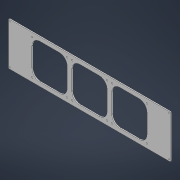
# Autodesk Inventor part: radiator_adapter_03
Saved by Autodesk Inventor 2022 (Build 260153000, 153)
## iProperties
Created: 2025-02-08
Part Number: radiator_adapter_03
Material: 一般
Document SubType Name: Modeling
Designer: gisen
Density: 1 g/cm^3
Appearance: 既定
Author: gisen
Autodesk Inventor part; units mm, degrees
ref_plane "YZ Plane" through (0, 0, 0) normal (1, 0, 0) x (0, 1, 0)
ref_plane "XZ Plane" through (0, 0, 0) normal (0, 1, 0) x (-1, 0, 0)
ref_plane "XY Plane" through (0, 0, 0) normal (0, 0, 1) x (1, 0, 0)
sketch "スケッチ1" plane through (0, 0, 0) normal (0, 0, 1) x (1, 0, 0)
  circle A0 centre (5, 125) radius 2.25 construction
  circle A1 centre (5, 5) radius 2.25 construction
  circle A2 centre (-473, 125) radius 2.25 construction
  circle A3 centre (-473, 5) radius 2.25 construction
  line L0 (-478, 130) -> (-478, 0) construction
  line L1 (10, 0) -> (10, 130) construction
  line L2 (10, 130) -> (-478, 130)
  line L3 (-478, 130) -> (-478, 0)
  line L4 (-478, 0) -> (10, 0)
  line L5 (10, 0) -> (10, 130)
  circle A4 centre (5, 125) radius 1.6
  circle A5 centre (5, 5) radius 1.6
  circle A6 centre (-473, 5) radius 1.6
  circle A7 centre (-473, 125) radius 1.6
  line L6 (10, 65) -> (-478, 65) construction
  line L7 (-205, 118) -> (-263, 118)
  line L8 (-287, 94) -> (-287, 36)
  line L9 (-263, 12) -> (-205, 12)
  line L10 (-181, 36) -> (-181, 94)
  arc A8 (-181, 94) -> (-205, 118) centre (-205, 94) ccw
  arc A9 (-205, 12) -> (-181, 36) centre (-205, 36) ccw
  arc A10 (-287, 36) -> (-263, 12) centre (-263, 36) ccw
  arc A11 (-263, 118) -> (-287, 94) centre (-263, 94) ccw
  line L11 (-174, 125) -> (-294, 125) construction
  line L12 (-294, 125) -> (-294, 5) construction
  line L13 (-294, 5) -> (-174, 5) construction
  line L14 (-174, 5) -> (-174, 125) construction
  line L15 (-181.6, 117.4) -> (-286.4, 117.4) construction
  line L16 (-286.4, 117.4) -> (-286.4, 12.6) construction
  line L17 (-286.4, 12.6) -> (-181.6, 12.6) construction
  line L18 (-181.6, 12.6) -> (-181.6, 117.4) construction
  circle A12 centre (-181.6, 117.4) radius 2.25
  circle A13 centre (-181.6, 12.6) radius 2.25
  circle A14 centre (-286.4, 12.6) radius 2.25
  circle A15 centre (-286.4, 117.4) radius 2.25
  circle A16 centre (-301.6, 117.4) radius 2.25
  arc A17 (-301, 94) -> (-325, 118) centre (-325, 94) ccw
  line L19 (-301, 36) -> (-301, 94)
  arc A18 (-325, 12) -> (-301, 36) centre (-325, 36) ccw
  circle A19 centre (-301.6, 12.6) radius 2.25
  line L20 (-383, 12) -> (-325, 12)
  arc A20 (-407, 36) -> (-383, 12) centre (-383, 36) ccw
  circle A21 centre (-406.4, 12.6) radius 2.25
  line L21 (-407, 94) -> (-407, 36)
  circle A22 centre (-406.4, 117.4) radius 2.25
  arc A23 (-383, 118) -> (-407, 94) centre (-383, 94) ccw
  line L22 (-325, 118) -> (-383, 118)
  circle A24 centre (-61.6, 117.4) radius 2.25
  arc A25 (-61, 94) -> (-85, 118) centre (-85, 94) ccw
  line L23 (-61, 36) -> (-61, 94)
  arc A26 (-85, 12) -> (-61, 36) centre (-85, 36) ccw
  circle A27 centre (-61.6, 12.6) radius 2.25
  line L24 (-143, 12) -> (-85, 12)
  arc A28 (-167, 36) -> (-143, 12) centre (-143, 36) ccw
  circle A29 centre (-166.4, 12.6) radius 2.25
  line L25 (-167, 94) -> (-167, 36)
  circle A30 centre (-166.4, 117.4) radius 2.25
  arc A31 (-143, 118) -> (-167, 94) centre (-143, 94) ccw
  line L26 (-85, 118) -> (-143, 118)
  circle A32 centre (-181.6, 117.4) radius 2.25
  arc A33 (-181, 94) -> (-205, 118) centre (-205, 94) ccw
  line L27 (-181, 36) -> (-181, 94)
  arc A34 (-205, 12) -> (-181, 36) centre (-205, 36) ccw
  circle A35 centre (-181.6, 12.6) radius 2.25
  line L28 (-263, 12) -> (-205, 12)
  arc A36 (-287, 36) -> (-263, 12) centre (-263, 36) ccw
  circle A37 centre (-286.4, 12.6) radius 2.25
  line L29 (-287, 94) -> (-287, 36)
  circle A38 centre (-286.4, 117.4) radius 2.25
  arc A39 (-263, 118) -> (-287, 94) centre (-263, 94) ccw
  line L30 (-205, 118) -> (-263, 118)
  point P0 (0, 0)
  point P1 (-234, 65)
  point P2 (-287, 12)
  point P3 (-287, 118)
  point P4 (-181, 12)
  point P5 (-287, 65)
  point P6 (-294, 65)
  point P7 (-234, 12)
  point P8 (-234, 5)
  point P9 (-234, 118)
  point P10 (-181, 65)
  point P11 (-174, 65)
  point P12 (-181.6, 65)
  point P13 (-234, 125)
  point P14 (-234, 117.4)
  point P15 (-301, 12)
  point P16 (-301, 65)
  point P17 (-407, 12)
  point P18 (-354, 12)
  point P19 (-407, 118)
  point P20 (-407, 65)
  point P21 (-354, 118)
  point P22 (-61, 12)
  point P23 (-61, 65)
  point P24 (-167, 12)
  point P25 (-114, 12)
  point P26 (-167, 118)
  point P27 (-167, 65)
  point P28 (-114, 118)
  point P29 (-181, 12)
  point P30 (-181, 65)
  point P31 (-287, 12)
  point P32 (-234, 12)
  point P33 (-287, 118)
  point P34 (-287, 65)
  point P35 (-234, 118)
  dimension "d0" = 3.2
  dimension "d1" = 106
  dimension "d2" = 106
  dimension "d3" = 24
  dimension "d4" = 120
  dimension "d5" = 120
  dimension "d6" = 104.8
  dimension "d7" = 104.8
  dimension "d8" = 4.5
  dimension "d11" = 120
  dimension "d14" = 120
  constraints: 58 end point, 36 centre point, 32 point on circle, 24 point on line, 13 midpoint, 9 equal radius, 8 coincident, 8 parallel, 8 tangent, 6 horizontal, 4 perpendicular, 3 horizontal alignment, 3 vertical alignment, 105 other
  measures "d0" diameter of A4
  measures "d1" distance of point (-181, 12) point (-287, 12)
  measures "d2" distance of point (-287, 12) point (-287, 118)
  measures "d3" radius of A8
  measures "d4" distance of L11.end L12.end
  measures "d5" distance of L12.end L13.end
  measures "d6" distance of L17.end L16.end
  measures "d7" distance of L17.end L15.start
  measures "d8" diameter of A12
  measures "d11" distance of A12.centre A16.centre
  measures "d14" distance of A12.centre A24.centre
extrude "押し出し1" add sketch "スケッチ1" along normal blind 3
sketch "スケッチ2" plane through (0, 0, 3) normal (0, 0, 1) x (1, 0, 0)
  line L0 (-478, 130) -> (-478, 0) projected
  line L1 (-478, 0) -> (10, 0) projected
  line L2 (10, 0) -> (10, 130) projected
  line L3 (10, 130) -> (-478, 130) projected
  circle A0 centre (-286.4, 117.4) radius 2.25 projected
  arc A1 (-263, 118) -> (-287, 94) centre (-263, 94) ccw projected
  line L4 (-263, 118) -> (-205, 118) projected
  arc A2 (-181, 94) -> (-205, 118) centre (-205, 94) ccw projected
  line L5 (-181, 94) -> (-181, 36) projected
  arc A3 (-205, 12) -> (-181, 36) centre (-205, 36) ccw projected
  line L6 (-205, 12) -> (-263, 12) projected
  arc A4 (-287, 36) -> (-263, 12) centre (-263, 36) ccw projected
  line L7 (-287, 36) -> (-287, 94) projected
  circle A5 centre (-473, 125) radius 1.6 projected
  circle A6 centre (-473, 5) radius 1.6 projected
  circle A7 centre (5, 5) radius 1.6 projected
  circle A8 centre (5, 125) radius 1.6 projected
  circle A9 centre (-181.6, 117.4) radius 2.25 projected
  circle A10 centre (-181.6, 12.6) radius 2.25 projected
  circle A11 centre (-286.4, 12.6) radius 2.25 projected
  circle A12 centre (-166.4, 117.4) radius 2.25 projected
  circle A13 centre (-166.4, 12.6) radius 2.25 projected
  circle A14 centre (-61.6, 12.6) radius 2.25 projected
  line L8 (-61, 94) -> (-61, 36) projected
  arc A15 (-85, 12) -> (-61, 36) centre (-85, 36) ccw projected
  line L9 (-85, 12) -> (-143, 12) projected
  arc A16 (-167, 36) -> (-143, 12) centre (-143, 36) ccw projected
  line L10 (-167, 36) -> (-167, 94) projected
  arc A17 (-143, 118) -> (-167, 94) centre (-143, 94) ccw projected
  line L11 (-143, 118) -> (-85, 118) projected
  arc A18 (-61, 94) -> (-85, 118) centre (-85, 94) ccw projected
  circle A19 centre (-61.6, 117.4) radius 2.25 projected
  circle A20 centre (-406.4, 117.4) radius 2.25 projected
  circle A21 centre (-406.4, 12.6) radius 2.25 projected
  circle A22 centre (-301.6, 12.6) radius 2.25 projected
  line L12 (-301, 94) -> (-301, 36) projected
  arc A23 (-325, 12) -> (-301, 36) centre (-325, 36) ccw projected
  line L13 (-325, 12) -> (-383, 12) projected
  arc A24 (-407, 36) -> (-383, 12) centre (-383, 36) ccw projected
  line L14 (-407, 36) -> (-407, 94) projected
  arc A25 (-383, 118) -> (-407, 94) centre (-383, 94) ccw projected
  line L15 (-383, 118) -> (-325, 118) projected
  arc A26 (-301, 94) -> (-325, 118) centre (-325, 94) ccw projected
  circle A27 centre (-301.6, 117.4) radius 2.25 projected
  line L16 (-477.9, 129.9) -> (-477.9, 0.1)
  line L17 (-477.9, 0.1) -> (9.9, 0.1)
  line L18 (9.9, 0.1) -> (9.9, 129.9)
  line L19 (9.9, 129.9) -> (-477.9, 129.9)
  point P0 (0, 0)
  dimension "d19" = 0.1
  constraints: 8 end point, 3 other
  measures "d19" distance between parallel lines of L3 L19
extrude "押し出し2" cut sketch "スケッチ2" against normal through all contours L3 L2 L1 L0
fillet "フィレット1" radius 2 4 edges at (-477.9, 129.9, 1.5) (-477.9, 0.1, 1.5) (9.9, 0.1, 1.5) (9.9, 129.9, 1.5)
equation "\"d5\" = d4"
equation "\"d7\" = d6"
